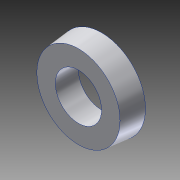
# Autodesk Inventor part: kop
Saved by Autodesk Inventor 2015 (Build 190159000, 159)
## iProperties
Created: 2016-01-04
Part Number: kop
Material: Generic
Document SubType Name: Modeling
Designer: david
Density: 1 g/cm^3
Appearance: Aluminum - Flat
Author: david
Autodesk Inventor part; units mm, degrees
ref_plane "YZ Plane" through (0, 0, 0) normal (1, 0, 0) x (0, 1, 0)
ref_plane "XZ Plane" through (0, 0, 0) normal (0, 1, 0) x (-1, 0, 0)
ref_plane "XY Plane" through (0, 0, 0) normal (0, 0, 1) x (1, 0, 0)
sketch "Sketch1" plane through (0, 0, 0) normal (0, 1, 0) x (-1, 0, 0)
  circle A0 centre (-3.2101, 3.6478) radius 9.5
  point P0 (0, 0)
  dimension "d0" = 19
  constraints: 1 centre point
  measures "d0" diameter of A0
extrude "Extrusion1" add sketch "Sketch1" along normal blind 5
chamfer "Chamfer1" distance 0.5 distance2 5 1 edges at (12.7101, 0, 3.6478) measured on face at (12.2101, 0, 3.6478)
sketch "Sketch2" plane through (3.2101, 0, 3.6478) normal (0, -1, 0) x (1, 0, 0)
  circle A0 centre (0, 0) radius 5
  point P0 (-3.2101, -3.6478)
  dimension "d6" = 10
  constraints: 1 centre point
  measures "d6" diameter of A0
extrude "Extrusion2" cut sketch "Sketch2" against normal blind 5
body "Solid1"
